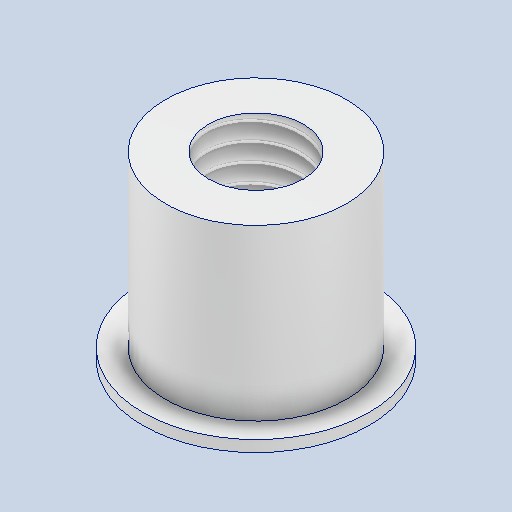
# Autodesk Inventor part: Návarek M5
Saved by Autodesk Inventor 2023 (Build 270158000, 158)
## iProperties
Created: 2023-03-26
Part Number: Návarek M5
Material: Aluminum 6061
Document SubType Name: Modeling
Designer: lukyv
Density: 2.7 g/cm^3
Appearance: Aluminum - Flat
Mass: 0.843353 g
Surface Area: 4.60243 cm^2
Volume: 0.312353 cm^3
Author: lukyv
Autodesk Inventor part; units mm, degrees
ref_plane "YZ Plane" through (0, 0, 0) normal (1, 0, 0) x (0, 1, 0)
ref_plane "XZ Plane" through (0, 0, 0) normal (0, 1, 0) x (-1, 0, 0)
ref_plane "XY Plane" through (0, 0, 0) normal (0, 0, 1) x (1, 0, 0)
sketch "Sketch1" plane through (0, 0, 0) normal (0, 1, 0) x (-1, 0, 0)
  circle A0 centre (0, 0) radius 2.1
  circle A1 centre (0, 0) radius 4
  circle A2 centre (0, 0) radius 5
  dimension "d0" = 4.2
  dimension "d1" = 8
  dimension "d2" = 10
  constraints: 3 centre point, 3 coincident
  measures "d0" diameter of A0
  measures "d1" diameter of A1
  measures "d2" diameter of A2
extrude "Extrusion1" add sketch "Sketch1" along normal blind 8 contours A1
extrude "Extrusion2" add sketch "Sketch1" along normal blind 0.5
thread "Thread1" size "M5x0.8" class "6H" standard "ANSI Metric M Profile" full length
body "Solid1"
